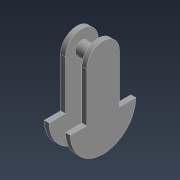
# Autodesk Inventor part: P015-Vilbrequin
Saved by Autodesk Inventor 2021.3 (Build 253353000, 353)
## iProperties
Created: 2022-04-01
Part Number: P015-Vilbrequin
Material: Générique
Document SubType Name: Modeling
Designer: remi
Density: 1 g/cm^3
Appearance: Par défaut
Author: remi
Autodesk Inventor part; units mm, degrees
ref_plane "YZ Plane" through (0, 0, 0) normal (1, 0, 0) x (0, 1, 0)
ref_plane "XZ Plane" through (0, 0, 0) normal (0, 1, 0) x (-1, 0, 0)
ref_plane "XY Plane" through (0, 0, 0) normal (0, 0, 1) x (1, 0, 0)
sketch "Sketch2" plane through (0, 0, 0) normal (1, 0, 0) x (0, 1, 0)
  arc A0 (-20, 0) -> (20, 0) centre (0, 0) ccw
  line L0 (-20, 0) -> (-10, 0)
  line L1 (-10, 0) -> (-10, 30)
  line L2 (20, 0) -> (10, 0)
  line L3 (10, 0) -> (10, 30)
  arc A1 (10, 30) -> (-10, 30) centre (0, 30) ccw
  dimension "d1" = 20
  dimension "d2" = 30
  dimension "d3" = 20
  constraints: 8 end point, 4 horizontal alignment, 4 point on circle, 2 centre point, 2 horizontal, 2 perpendicular, 1 coincident, 1 collinear
  measures "d1" distance between parallel lines of L3 L1
  measures "d2" distance of L2.end L3.end
  measures "d3" radius of A0
extrude "Extrusion1" add sketch "Sketch2" along normal blind 3
sketch "Sketch3" plane through (3, 0, 0) normal (1, 0, 0) x (0, 0, -1)
  arc A0 (0, -20) -> (0, 20) centre (0, 0) ccw construction
  line L0 (0, 20) -> (0, 10) construction
  line L1 (0, 10) -> (-30, 10) construction
  arc A1 (-30, 10) -> (-30, -10) centre (-30, 0) ccw construction
  line L2 (-30, -10) -> (0, -10) construction
  line L3 (0, -10) -> (0, -20) construction
  circle A2 centre (-30, 0) radius 4
  dimension "d6" = 8
  constraints: 1 centre point, 1 coincident
  measures "d6" diameter of A2
extrude "Extrusion2" add sketch "Sketch3" along normal blind 10
sketch "Sketch4" plane through (13, 0, 30) normal (1, 0, 0) x (0, 0, -1)
  circle A0 centre (0, 0) radius 4 projected
  arc A1 (30, -20) -> (30, 20) centre (30, 0) ccw projected
  line L0 (30, 20) -> (30, 10) projected
  line L1 (30, 10) -> (0, 10) projected
  arc A2 (0, 10) -> (0, -10) centre (0, 0) ccw projected
  line L2 (0, -10) -> (30, -10) projected
  line L3 (30, -10) -> (30, -20) projected
extrude "Extrusion3" add sketch "Sketch4" along normal blind 3 contours A0 | L3 L2 A2 L1 L0 A1
body "Solid1"
